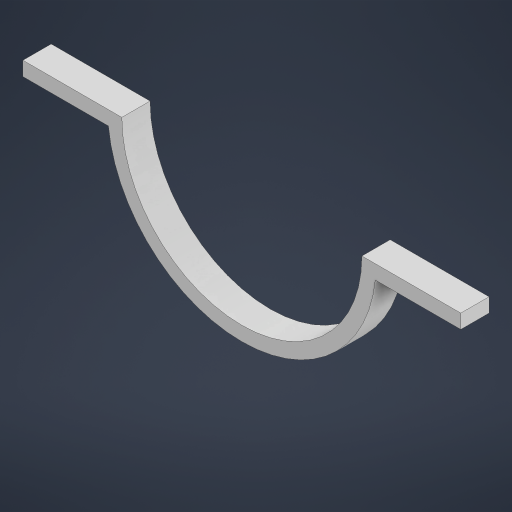
# Autodesk Inventor part: Part3
Saved by Autodesk Inventor 2023 (Build 270158030, 158C)
## iProperties
Created: 2023-02-03
Part Number: Part3
Material: Generic
Document SubType Name: Modeling
Designer: Monster
Density: 1 g/cm^3
Appearance: Default
Author: Monster
Autodesk Inventor part; units mm, degrees
ref_plane "YZ Plane" through (0, 0, 0) normal (1, 0, 0) x (0, 1, 0)
ref_plane "XZ Plane" through (0, 0, 0) normal (0, 1, 0) x (-1, 0, 0)
ref_plane "XY Plane" through (0, 0, 0) normal (0, 0, 1) x (1, 0, 0)
sketch "Sketch1" plane through (0, 0, 0) normal (0, 0, 1) x (1, 0, 0)
  arc A0 (-8.5, 0) -> (8.5, 0) centre (0, 0) ccw
  arc A1 (-9.5, 0) -> (9.5, 0) centre (0, 0) ccw
  line L0 (-8.5, 0) -> (-15.5, 0)
  line L1 (8.5, 0) -> (15.5, 0)
  line L2 (15.5, 0) -> (15.5, -1)
  line L3 (15.5, -1) -> (9.4472, -1)
  line L4 (-15.5, 0) -> (-15.5, -1)
  line L5 (-15.5, -1) -> (-9.4472, -1)
  dimension "d0" = 8.5
  dimension "d1" = 9.5
  dimension "d2" = 7
  dimension "d3" = 7
  dimension "d4" = 1
  dimension "d5" = 1
  constraints: 12 end point, 6 point on circle, 3 perpendicular, 2 centre point, 2 coincident, 2 horizontal, 1 vertical
  measures "d0" radius of A0
  measures "d1" radius of A1
  measures "d2" distance of L0.start L0.end
  measures "d3" distance of L1.start L1.end
  measures "d4" distance of L1.end L2.end
  measures "d5" distance of L0.end L4.end
extrude "Extrusion1" add sketch "Sketch1" along normal blind 2
body "Solid1"
